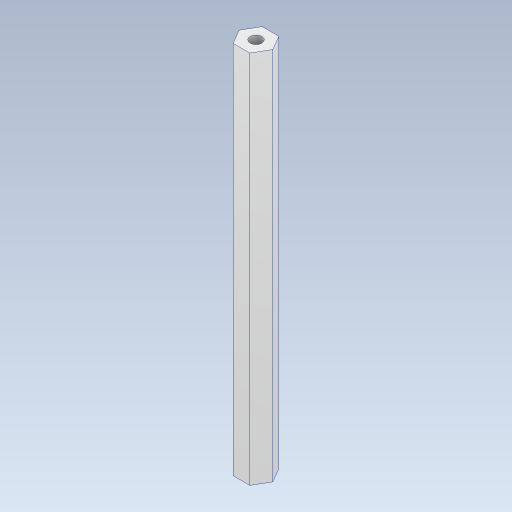
# Autodesk Inventor part: INDEX_009_6inHex
Saved by Autodesk Inventor 2024 (Build 280153000, 153)
## iProperties
Created: 2024-08-09
Part Number: INDEX_009_6inHex
Material: Aluminum 6061
Document SubType Name: Modeling
Designer: Oscar
Density: 2.7 g/cm^3
Appearance: Aluminum - Flat
Author: Oscar
Autodesk Inventor part; units mm, degrees
ref_plane "YZ Plane" through (0, 0, 0) normal (1, 0, 0) x (0, 1, 0)
ref_plane "XZ Plane" through (0, 0, 0) normal (0, 1, 0) x (-1, 0, 0)
ref_plane "XY Plane" through (0, 0, 0) normal (0, 0, 1) x (1, 0, 0)
sketch "Sketch1" plane through (0, 0, 0) normal (0, 1, 0) x (-1, 0, 0)
  line L0 (-7.3323, 0) -> (-3.6662, 6.35)
  line L1 (-3.6662, 6.35) -> (3.6662, 6.35)
  line L2 (3.6662, 6.35) -> (7.3323, 0)
  line L3 (7.3323, 0) -> (3.6662, -6.35)
  line L4 (3.6662, -6.35) -> (-3.6662, -6.35)
  line L5 (-3.6662, -6.35) -> (-7.3323, 0)
  point P0 (0, 0)
  point P1 (0, 0)
  point P2 (-5.4993, 3.175)
  dimension "d0" = 12.7
  constraints: 12 end point, 1 coincident, 1 horizontal, 1 midpoint, 13 other
  measures "d0" distance from line of L3 point (-5.499, 3.175)
extrude "Extrusion1" add sketch "Sketch1" along normal blind 163.576
sketch "Sketch2" plane through (0, 163.576, 0) normal (0, 1, 0) x (1, 0, 0)
  circle A0 centre (0, 0) radius 2.5527
  dimension "d3" = 5.1054
  constraints: 1 centre point, 1 coincident
  measures "d3" diameter of A0
extrude "Extrusion2" cut sketch "Sketch2" against normal blind 25.4
body "Solid1"
